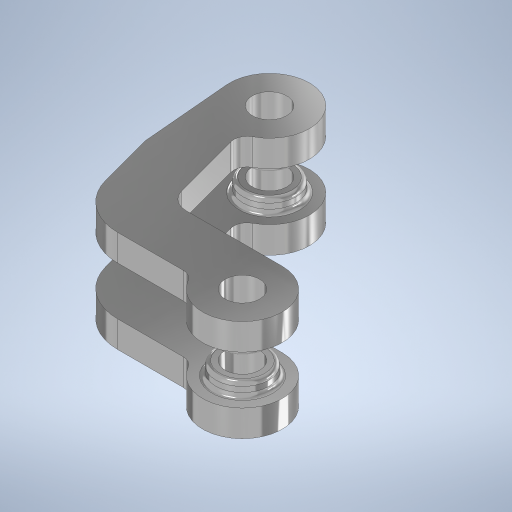
# Autodesk Inventor part: Levers
Saved by Autodesk Inventor 2024 (Build 280153000, 153)
## iProperties
Created: 2007-06-13
Part Number: Levers
Material: Steel
Description: Levers
Document SubType Name: Modeling
Designer: G.K.
Authority: Design by UAB Čeli APS
Mass: 1.86899 g
Surface Area: 4.18262 cm^2
Volume: 0.238088 cm^3
Density: 7.85 g/cm^3
Appearance: Chrome - Polished
Mase: 0.00186899
Autodesk Inventor part; units mm, degrees
ref_plane "YZ Plane" through (0, 0, 0) normal (1, 0, 0) x (0, 1, 0)
ref_plane "XZ Plane" through (0, 0, 0) normal (0, 1, 0) x (-1, 0, 0)
sketch "Sketch1" plane through (0, 0, 0) normal (0, 0, 1) x (1, 0, 0)
  line L0 (0, 0) -> (-10.9545, 13) construction
  line L1 (-18.0822, 0) -> (7.7948, 0) projected
  circle A0 centre (0, 0) radius 1.3
  circle A1 centre (-10.9545, 13) radius 1.3
  arc A2 (-9.5657, 10.3408) -> (-13.943, 12.7385) centre (-10.9545, 13) ccw
  arc A3 (-2.5981, -1.5) -> (0, 3) centre (0, 0) ccw
  line L2 (-13.943, 12.7385) -> (-13.3535, 6)
  line L3 (-13.3535, 6) -> (-12.2722, 1.9647)
  line L4 (-10.0686, 9.1956) -> (-8.7064, 4.1118)
  line L5 (-7.2575, 3) -> (0, 3)
  line L6 (-3.4641, -1) -> (-8.4085, -1)
  arc A4 (-9.5657, 10.3408) -> (-10.0686, 9.1956) centre (-9.1027, 9.4544) ccw
  arc A5 (-8.7064, 4.1118) -> (-7.2575, 3) centre (-7.2575, 4.5) ccw
  arc A6 (-12.2722, 1.9647) -> (-8.4085, -1) centre (-8.4085, 3) ccw
  arc A7 (-2.5981, -1.5) -> (-3.4641, -1) centre (-3.4641, -2) ccw
  dimension "d0" = 17
  dimension "d2" = 2.6
  dimension "d4" = 4
  dimension "d5" = 6
  dimension "d6" = 4
  dimension "d7" = 105
  dimension "d13" = 6
  dimension "d15" = 1
  dimension "d16" = 1.5
  dimension "d17" = 4
  dimension "d18" = 1
  dimension "d25" = 14
  dimension "d27" = 10
  constraints: 13 end point, 12 point on circle, 10 tangent, 8 centre point, 4 coincident, 2 equal radius, 2 parallel, 1 horizontal
  measures "d0" distance of L0.start L0.end
  measures "d2" diameter of A1
  measures "d4" distance between parallel lines of L4 L3
  measures "d5" diameter of A2
  measures "d6" distance between parallel lines of L6 L5
  measures "d7" angle of L4 L5
  measures "d13" distance from line of L1 L2.end
  measures "d15" radius of A4
  measures "d16" radius of A5
  measures "d17" radius of A6
  measures "d18" radius of A7
  measures "d25" distance from line of A1.centre L6
  measures "d27" angle of L3 L2
extrude "Extrusion1" add sketch "Sketch1" along normal blind 2 contours A6 L3 L2 A2 A4 L4 A5 L5 A3 L1 A0 | L1 A0 A3 A7 L6 A6
sketch "Sketch2" plane through (0, 0, 2) normal (0, 0, 1) x (1, 0, 0)
  circle A0 centre (-10.9545, 13) radius 1.3 projected
  circle A1 centre (0, 0) radius 1.3 projected
  arc A2 (-9.5657, 10.3408) -> (-13.943, 12.7385) centre (-10.9545, 13) ccw projected
  arc A3 (-2.5981, -1.5) -> (0, 3) centre (0, 0) ccw projected
  circle A4 centre (-10.9545, 13) radius 2
  circle A5 centre (0, 0) radius 2
  dimension "d21" = 0.7
  constraints: 2 centre point, 2 coincident, 1 equal radius
  measures "d21" radial gap between concentric circles of A4 A0
extrude "Extrusion2" add sketch "Sketch2" along normal blind 1
fillet "Fillet1" radius 0.3 4 edges at (-2, 0, 2) (-12.9545, 13, 2) (-12.9545, 13, 3) (-2, 0, 3)
ref_plane "Work Plane1" through (0, 0, 3.825) normal (0, 0, 1) x (1, 0, 0)
mirror "Mirror1" about plane through (0, 0, 3.825) normal (0, 0, 1)
body "Solid1"
